Autodesk Fusion 360 part; units mm, degrees
(part 6 of 9)
  line L309 (-65.5897, 101.2894) -> (-69.9199, 98.7894)
  line L310 (-69.9199, 98.7894) -> (-74.25, 101.2894)
  line L311 (-74.25, 101.2894) -> (-74.25, 106.2894)
  line L312 (-48.8494, 97.4904) -> (-44.5192, 99.9904)
  line L313 (-44.5192, 99.9904) -> (-40.1891, 97.4904)
  line L314 (-40.1891, 97.4904) -> (-40.1891, 92.4904)
  line L315 (-40.1891, 92.4904) -> (-44.5192, 89.9904)
  line L316 (-44.5192, 89.9904) -> (-48.8494, 92.4904)
  line L317 (-48.8494, 92.4904) -> (-48.8494, 97.4904)
  line L318 (-23.4487, 88.6913) -> (-19.1186, 91.1913)
  line L319 (-19.1186, 91.1913) -> (-14.7885, 88.6913)
  line L320 (-14.7885, 88.6913) -> (-14.7885, 83.6913)
  line L321 (-14.7885, 83.6913) -> (-19.1186, 81.1913)
  line L322 (-19.1186, 81.1913) -> (-23.4487, 83.6913)
  line L323 (-23.4487, 83.6913) -> (-23.4487, 88.6913)
  line L324 (-64.0897, 88.6913) -> (-59.7596, 91.1913)
  line L325 (-59.7596, 91.1913) -> (-55.4295, 88.6913)
  line L326 (-55.4295, 88.6913) -> (-55.4295, 83.6913)
  line L327 (-55.4295, 83.6913) -> (-59.7596, 81.1913)
  line L328 (-59.7596, 81.1913) -> (-64.0897, 83.6913)
  line L329 (-64.0897, 83.6913) -> (-64.0897, 88.6913)
  line L330 (-38.6891, 79.8923) -> (-34.359, 82.3923)
  line L331 (-34.359, 82.3923) -> (-30.0289, 79.8923)
  line L332 (-30.0289, 79.8923) -> (-30.0289, 74.8923)
  line L333 (-30.0289, 74.8923) -> (-34.359, 72.3923)
  line L334 (-34.359, 72.3923) -> (-38.6891, 74.8923)
  line L335 (-38.6891, 74.8923) -> (-38.6891, 79.8923)
  line L336 (-79.3301, 79.8923) -> (-75, 82.3923)
  line L337 (-75, 82.3923) -> (-70.6699, 79.8923)
  line L338 (-70.6699, 79.8923) -> (-70.6699, 74.8923)
  line L339 (-70.6699, 74.8923) -> (-75, 72.3923)
  line L340 (-75, 72.3923) -> (-79.3301, 74.8923)
  line L341 (-79.3301, 74.8923) -> (-79.3301, 79.8923)
  line L342 (-53.9295, 71.0933) -> (-49.5994, 73.5933)
  line L343 (-49.5994, 73.5933) -> (-45.2692, 71.0933)
  line L344 (-45.2692, 71.0933) -> (-45.2692, 66.0933)
  line L345 (-45.2692, 66.0933) -> (-49.5994, 63.5933)
  line L346 (-49.5994, 63.5933) -> (-53.9295, 66.0933)
  line L347 (-53.9295, 66.0933) -> (-53.9295, 71.0933)
  line L348 (-28.5289, 62.2942) -> (-24.1987, 64.7942)
  line L349 (-24.1987, 64.7942) -> (-19.8686, 62.2942)
  line L350 (-19.8686, 62.2942) -> (-19.8686, 57.2942)
  line L351 (-19.8686, 57.2942) -> (-24.1987, 54.7942)
  line L352 (-24.1987, 54.7942) -> (-28.5289, 57.2942)
  line L353 (-28.5289, 57.2942) -> (-28.5289, 62.2942)
  line L354 (-69.1699, 62.2942) -> (-64.8397, 64.7942)
  line L355 (-64.8397, 64.7942) -> (-60.5096, 62.2942)
  line L356 (-60.5096, 62.2942) -> (-60.5096, 57.2942)
  line L357 (-60.5096, 57.2942) -> (-64.8397, 54.7942)
  line L358 (-64.8397, 54.7942) -> (-69.1699, 57.2942)
  line L359 (-69.1699, 57.2942) -> (-69.1699, 62.2942)
  line L360 (-43.7692, 53.4952) -> (-39.4391, 55.9952)
  line L361 (-39.4391, 55.9952) -> (-35.109, 53.4952)
  line L362 (-35.109, 53.4952) -> (-35.109, 48.4952)
  line L363 (-35.109, 48.4952) -> (-39.4391, 45.9952)
  line L364 (-39.4391, 45.9952) -> (-43.7692, 48.4952)
  line L365 (-43.7692, 48.4952) -> (-43.7692, 53.4952)
  line L366 (-18.3686, 44.6962) -> (-14.0385, 47.1962)
  line L367 (-14.0385, 47.1962) -> (-9.7083, 44.6962)
  line L368 (-9.7083, 44.6962) -> (-9.7083, 39.6962)
  line L369 (-9.7083, 39.6962) -> (-14.0385, 37.1962)
  line L370 (-14.0385, 37.1962) -> (-18.3686, 39.6962)
  line L371 (-18.3686, 39.6962) -> (-18.3686, 44.6962)
  line L372 (-59.0096, 44.6962) -> (-54.6795, 47.1962)
  line L373 (-54.6795, 47.1962) -> (-50.3494, 44.6962)
  line L374 (-50.3494, 44.6962) -> (-50.3494, 39.6962)
  line L375 (-50.3494, 39.6962) -> (-54.6795, 37.1962)
  line L376 (-54.6795, 37.1962) -> (-59.0096, 39.6962)
  line L377 (-59.0096, 39.6962) -> (-59.0096, 44.6962)
  line L378 (-33.609, 35.8971) -> (-29.2789, 38.3971)
  line L379 (-29.2789, 38.3971) -> (-24.9487, 35.8971)
  line L380 (-24.9487, 35.8971) -> (-24.9487, 30.8971)
  line L381 (-24.9487, 30.8971) -> (-29.2789, 28.3971)
  line L382 (-29.2789, 28.3971) -> (-33.609, 30.8971)
  line L383 (-33.609, 30.8971) -> (-33.609, 35.8971)
  line L384 (-74.25, 35.8971) -> (-69.9199, 38.3971)
  line L385 (-69.9199, 38.3971) -> (-65.5897, 35.8971)
  line L386 (-65.5897, 35.8971) -> (-65.5897, 30.8971)
  line L387 (-65.5897, 30.8971) -> (-69.9199, 28.3971)
  line L388 (-69.9199, 28.3971) -> (-74.25, 30.8971)
  line L389 (-74.25, 30.8971) -> (-74.25, 35.8971)
  line L390 (-48.8494, 27.0981) -> (-44.5192, 29.5981)
  line L391 (-44.5192, 29.5981) -> (-40.1891, 27.0981)
  line L392 (-40.1891, 27.0981) -> (-40.1891, 22.0981)
  line L393 (-40.1891, 22.0981) -> (-44.5192, 19.5981)
  line L394 (-44.5192, 19.5981) -> (-48.8494, 22.0981)
  line L395 (-48.8494, 22.0981) -> (-48.8494, 27.0981)
  line L396 (-23.4487, 18.299) -> (-19.1186, 20.799)
  line L397 (-19.1186, 20.799) -> (-14.7885, 18.299)
  line L398 (-14.7885, 18.299) -> (-14.7885, 13.299)
  line L399 (-14.7885, 13.299) -> (-19.1186, 10.799)
  line L400 (-19.1186, 10.799) -> (-23.4487, 13.299)
  line L401 (-23.4487, 13.299) -> (-23.4487, 18.299)
  line L402 (-64.0897, 18.299) -> (-59.7596, 20.799)
  line L403 (-59.7596, 20.799) -> (-55.4295, 18.299)
  line L404 (-55.4295, 18.299) -> (-55.4295, 13.299)
  line L405 (-55.4295, 13.299) -> (-59.7596, 10.799)
  line L406 (-59.7596, 10.799) -> (-64.0897, 13.299)
  line L407 (-64.0897, 13.299) -> (-64.0897, 18.299)
  line L408 (-53.9295, 18.299) -> (-49.5994, 20.799)
  line L409 (-49.5994, 20.799) -> (-45.2692, 18.299)
  line L410 (-45.2692, 18.299) -> (-45.2692, 13.299)
  line L411 (-45.2692, 13.299) -> (-49.5994, 10.799)
  line L412 (-49.5994, 10.799) -> (-53.9295, 13.299)
  line L413 (-53.9295, 13.299) -> (-53.9295, 18.299)
  line L414 (-79.3301, 27.0981) -> (-75, 29.5981)
  line L415 (-75, 29.5981) -> (-70.6699, 27.0981)
  line L416 (-70.6699, 27.0981) -> (-70.6699, 22.0981)
  line L417 (-70.6699, 22.0981) -> (-75, 19.5981)
  line L418 (-75, 19.5981) -> (-79.3301, 22.0981)
  line L419 (-79.3301, 22.0981) -> (-79.3301, 27.0981)
  line L420 (-38.6891, 27.0981) -> (-34.359, 29.5981)
  line L421 (-34.359, 29.5981) -> (-30.0289, 27.0981)
  line L422 (-30.0289, 27.0981) -> (-30.0289, 22.0981)
  line L423 (-30.0289, 22.0981) -> (-34.359, 19.5981)
  line L424 (-34.359, 19.5981) -> (-38.6891, 22.0981)
  line L425 (-38.6891, 22.0981) -> (-38.6891, 27.0981)
  line L426 (-64.0897, 35.8971) -> (-59.7596, 38.3971)
  line L427 (-59.7596, 38.3971) -> (-55.4295, 35.8971)
  line L428 (-55.4295, 35.8971) -> (-55.4295, 30.8971)
  line L429 (-55.4295, 30.8971) -> (-59.7596, 28.3971)
  line L430 (-59.7596, 28.3971) -> (-64.0897, 30.8971)
  line L431 (-64.0897, 30.8971) -> (-64.0897, 35.8971)
  line L432 (-23.4487, 35.8971) -> (-19.1186, 38.3971)
  line L433 (-19.1186, 38.3971) -> (-14.7885, 35.8971)
  line L434 (-14.7885, 35.8971) -> (-14.7885, 30.8971)
  line L435 (-14.7885, 30.8971) -> (-19.1186, 28.3971)
  line L436 (-19.1186, 28.3971) -> (-23.4487, 30.8971)
  line L437 (-23.4487, 30.8971) -> (-23.4487, 35.8971)
  line L438 (-48.8494, 44.6962) -> (-44.5192, 47.1962)
  line L439 (-44.5192, 47.1962) -> (-40.1891, 44.6962)
  line L440 (-40.1891, 44.6962) -> (-40.1891, 39.6962)
  line L441 (-40.1891, 39.6962) -> (-44.5192, 37.1962)
  line L442 (-44.5192, 37.1962) -> (-48.8494, 39.6962)
  line L443 (-48.8494, 39.6962) -> (-48.8494, 44.6962)
  line L444 (-74.25, 53.4952) -> (-69.9199, 55.9952)
  line L445 (-69.9199, 55.9952) -> (-65.5897, 53.4952)
  line L446 (-65.5897, 53.4952) -> (-65.5897, 48.4952)
  line L447 (-65.5897, 48.4952) -> (-69.9199, 45.9952)
  line L448 (-69.9199, 45.9952) -> (-74.25, 48.4952)
  line L449 (-74.25, 48.4952) -> (-74.25, 53.4952)
  line L450 (-33.609, 53.4952) -> (-29.2789, 55.9952)
  line L451 (-29.2789, 55.9952) -> (-24.9487, 53.4952)
  line L452 (-24.9487, 53.4952) -> (-24.9487, 48.4952)
  line L453 (-24.9487, 48.4952) -> (-29.2789, 45.9952)
  line L454 (-29.2789, 45.9952) -> (-33.609, 48.4952)
  line L455 (-33.609, 48.4952) -> (-33.609, 53.4952)
  line L456 (-59.0096, 62.2942) -> (-54.6795, 64.7942)
  line L457 (-54.6795, 64.7942) -> (-50.3494, 62.2942)
  line L458 (-50.3494, 62.2942) -> (-50.3494, 57.2942)
  line L459 (-50.3494, 57.2942) -> (-54.6795, 54.7942)
  line L460 (-54.6795, 54.7942) -> (-59.0096, 57.2942)
  line L461 (-59.0096, 57.2942) -> (-59.0096, 62.2942)
  line L462 (-18.3686, 62.2942) -> (-14.0385, 64.7942)
  line L463 (-14.0385, 64.7942) -> (-9.7083, 62.2942)
  line L464 (-9.7083, 62.2942) -> (-9.7083, 57.2942)
  line L465 (-9.7083, 57.2942) -> (-14.0385, 54.7942)
  line L466 (-14.0385, 54.7942) -> (-18.3686, 57.2942)
  line L467 (-18.3686, 57.2942) -> (-18.3686, 62.2942)
  line L468 (-43.7692, 71.0933) -> (-39.4391, 73.5933)
  line L469 (-39.4391, 73.5933) -> (-35.109, 71.0933)
  line L470 (-35.109, 71.0933) -> (-35.109, 66.0933)
  line L471 (-35.109, 66.0933) -> (-39.4391, 63.5933)
  line L472 (-39.4391, 63.5933) -> (-43.7692, 66.0933)
  line L473 (-43.7692, 66.0933) -> (-43.7692, 71.0933)
  line L474 (-69.1699, 79.8923) -> (-64.8397, 82.3923)
  line L475 (-64.8397, 82.3923) -> (-60.5096, 79.8923)
  line L476 (-60.5096, 79.8923) -> (-60.5096, 74.8923)
  line L477 (-60.5096, 74.8923) -> (-64.8397, 72.3923)
  line L478 (-64.8397, 72.3923) -> (-69.1699, 74.8923)
  line L479 (-69.1699, 74.8923) -> (-69.1699, 79.8923)
  line L480 (-28.5289, 79.8923) -> (-24.1987, 82.3923)
  line L481 (-24.1987, 82.3923) -> (-19.8686, 79.8923)
  line L482 (-19.8686, 79.8923) -> (-19.8686, 74.8923)
  line L483 (-19.8686, 74.8923) -> (-24.1987, 72.3923)
  line L484 (-24.1987, 72.3923) -> (-28.5289, 74.8923)
  line L485 (-28.5289, 74.8923) -> (-28.5289, 79.8923)
  line L486 (-53.9295, 88.6913) -> (-49.5994, 91.1913)
  line L487 (-49.5994, 91.1913) -> (-45.2692, 88.6913)
  line L488 (-45.2692, 88.6913) -> (-45.2692, 83.6913)
  line L489 (-45.2692, 83.6913) -> (-49.5994, 81.1913)
  line L490 (-49.5994, 81.1913) -> (-53.9295, 83.6913)
  line L491 (-53.9295, 83.6913) -> (-53.9295, 88.6913)
  line L492 (-79.3301, 97.4904) -> (-75, 99.9904)
  line L493 (-75, 99.9904) -> (-70.6699, 97.4904)
  line L494 (-70.6699, 97.4904) -> (-70.6699, 92.4904)
  line L495 (-70.6699, 92.4904) -> (-75, 89.9904)
  line L496 (-75, 89.9904) -> (-79.3301, 92.4904)
  line L497 (-79.3301, 92.4904) -> (-79.3301, 97.4904)
  line L498 (-38.6891, 97.4904) -> (-34.359, 99.9904)
  line L499 (-34.359, 99.9904) -> (-30.0289, 97.4904)
  line L500 (-30.0289, 97.4904) -> (-30.0289, 92.4904)
  line L501 (-30.0289, 92.4904) -> (-34.359, 89.9904)
  line L502 (-34.359, 89.9904) -> (-38.6891, 92.4904)
  line L503 (-38.6891, 92.4904) -> (-38.6891, 97.4904)
  line L504 (-64.0897, 106.2894) -> (-59.7596, 108.7894)
  line L505 (-59.7596, 108.7894) -> (-55.4295, 106.2894)
  line L506 (-55.4295, 106.2894) -> (-55.4295, 101.2894)
  line L507 (-55.4295, 101.2894) -> (-59.7596, 98.7894)
  line L508 (-59.7596, 98.7894) -> (-64.0897, 101.2894)
  line L509 (-64.0897, 101.2894) -> (-64.0897, 106.2894)
  line L510 (-23.4487, 106.2894) -> (-19.1186, 108.7894)
  line L511 (-19.1186, 108.7894) -> (-14.7885, 106.2894)
  line L512 (-14.7885, 106.2894) -> (-14.7885, 101.2894)
  line L513 (-14.7885, 101.2894) -> (-19.1186, 98.7894)
  line L514 (-19.1186, 98.7894) -> (-23.4487, 101.2894)
  line L515 (-23.4487, 101.2894) -> (-23.4487, 106.2894)
  line L516 (-48.8494, 115.0885) -> (-44.5192, 117.5885)
  line L517 (-44.5192, 117.5885) -> (-40.1891, 115.0885)
  line L518 (-40.1891, 115.0885) -> (-40.1891, 110.0885)
  line L519 (-40.1891, 110.0885) -> (-44.5192, 107.5885)
  line L520 (-44.5192, 107.5885) -> (-48.8494, 110.0885)
  line L521 (-48.8494, 110.0885) -> (-48.8494, 115.0885)
  line L522 (-74.25, 123.8875) -> (-69.9199, 126.3875)
  line L523 (-69.9199, 126.3875) -> (-65.5897, 123.8875)
  line L524 (-65.5897, 123.8875) -> (-65.5897, 118.8875)
  line L525 (-65.5897, 118.8875) -> (-69.9199, 116.3875)
  line L526 (-69.9199, 116.3875) -> (-74.25, 118.8875)
  line L527 (-74.25, 118.8875) -> (-74.25, 123.8875)
  line L528 (-33.609, 123.8875) -> (-29.2789, 126.3875)
  line L529 (-29.2789, 126.3875) -> (-24.9487, 123.8875)
  line L530 (-24.9487, 123.8875) -> (-24.9487, 118.8875)
  line L531 (-24.9487, 118.8875) -> (-29.2789, 116.3875)
  line L532 (-29.2789, 116.3875) -> (-33.609, 118.8875)
  line L533 (-33.609, 118.8875) -> (-33.609, 123.8875)
  line L534 (-59.0096, 132.6865) -> (-54.6795, 135.1865)
  line L535 (-54.6795, 135.1865) -> (-50.3494, 132.6865)
  line L536 (-50.3494, 132.6865) -> (-50.3494, 127.6865)
  line L537 (-50.3494, 127.6865) -> (-54.6795, 125.1865)
  line L538 (-54.6795, 125.1865) -> (-59.0096, 127.6865)
  line L539 (-59.0096, 127.6865) -> (-59.0096, 132.6865)
  line L540 (-18.3686, 132.6865) -> (-14.0385, 135.1865)
  line L541 (-14.0385, 135.1865) -> (-9.7083, 132.6865)
  line L542 (-9.7083, 132.6865) -> (-9.7083, 127.6865)
  line L543 (-9.7083, 127.6865) -> (-14.0385, 125.1865)
  line L544 (-14.0385, 125.1865) -> (-18.3686, 127.6865)
  line L545 (-18.3686, 127.6865) -> (-18.3686, 132.6865)
  line L546 (-82, 0) -> (-7, 0)
  line L547 (-7, 0) -> (-7, 140)
  line L548 (-7, 140) -> (-82, 140)
  line L549 (-82, 140) -> (-82, 0)
  line L550 (-69.9199, 20.799) -> (-74.25, 18.299)
  line L551 (-74.25, 18.299) -> (-74.25, 13.299)
  line L552 (-74.25, 13.299) -> (-69.9199, 10.799)
  line L553 (-69.9199, 10.799) -> (-65.5897, 13.299)
  line L554 (-65.5897, 13.299) -> (-65.5897, 18.299)
  line L555 (-65.5897, 18.299) -> (-69.9199, 20.799)
  line L556 (-59.7596, 20.799) -> (-64.0897, 18.299)
  line L557 (-64.0897, 18.299) -> (-64.0897, 13.299)
  line L558 (-64.0897, 13.299) -> (-59.7596, 10.799)
  line L559 (-59.7596, 10.799) -> (-55.4295, 13.299)
  line L560 (-55.4295, 13.299) -> (-55.4295, 18.299)
  line L561 (-55.4295, 18.299) -> (-59.7596, 20.799)
  line L562 (-49.5994, 20.799) -> (-53.9295, 18.299)
  line L563 (-53.9295, 18.299) -> (-53.9295, 13.299)
  line L564 (-53.9295, 13.299) -> (-49.5994, 10.799)
  line L565 (-49.5994, 10.799) -> (-45.2692, 13.299)
  line L566 (-45.2692, 13.299) -> (-45.2692, 18.299)
  line L567 (-45.2692, 18.299) -> (-49.5994, 20.799)
  line L568 (-39.4391, 20.799) -> (-43.7692, 18.299)
  line L569 (-43.7692, 18.299) -> (-43.7692, 13.299)
  line L570 (-43.7692, 13.299) -> (-39.4391, 10.799)
  line L571 (-39.4391, 10.799) -> (-35.109, 13.299)
  line L572 (-35.109, 13.299) -> (-35.109, 18.299)
  line L573 (-35.109, 18.299) -> (-39.4391, 20.799)
  line L574 (-29.2789, 20.799) -> (-33.609, 18.299)
  line L575 (-33.609, 18.299) -> (-33.609, 13.299)
  line L576 (-33.609, 13.299) -> (-29.2789, 10.799)
  line L577 (-29.2789, 10.799) -> (-24.9487, 13.299)
  line L578 (-24.9487, 13.299) -> (-24.9487, 18.299)
  line L579 (-24.9487, 18.299) -> (-29.2789, 20.799)
  line L580 (-19.1186, 20.799) -> (-23.4487, 18.299)
  line L581 (-23.4487, 18.299) -> (-23.4487, 13.299)
  line L582 (-23.4487, 13.299) -> (-19.1186, 10.799)
  line L583 (-19.1186, 10.799) -> (-14.7885, 13.299)
  line L584 (-14.7885, 13.299) -> (-14.7885, 18.299)
  line L585 (-14.7885, 18.299) -> (-19.1186, 20.799)
  line L586 (-75, 29.5981) -> (-79.3301, 27.0981)
  line L587 (-79.3301, 27.0981) -> (-79.3301, 22.0981)
  line L588 (-79.3301, 22.0981) -> (-75, 19.5981)
  line L589 (-75, 19.5981) -> (-70.6699, 22.0981)
  line L590 (-70.6699, 22.0981) -> (-70.6699, 27.0981)
  line L591 (-70.6699, 27.0981) -> (-75, 29.5981)
  line L592 (-64.8397, 29.5981) -> (-69.1699, 27.0981)
  line L593 (-69.1699, 27.0981) -> (-69.1699, 22.0981)
  line L594 (-69.1699, 22.0981) -> (-64.8397, 19.5981)
  line L595 (-64.8397, 19.5981) -> (-60.5096, 22.0981)
  line L596 (-60.5096, 22.0981) -> (-60.5096, 27.0981)
  line L597 (-60.5096, 27.0981) -> (-64.8397, 29.5981)
  line L598 (-54.6795, 29.5981) -> (-59.0096, 27.0981)
  line L599 (-59.0096, 27.0981) -> (-59.0096, 22.0981)
  line L600 (-59.0096, 22.0981) -> (-54.6795, 19.5981)
  line L601 (-54.6795, 19.5981) -> (-50.3494, 22.0981)
  line L602 (-50.3494, 22.0981) -> (-50.3494, 27.0981)
  line L603 (-50.3494, 27.0981) -> (-54.6795, 29.5981)
  line L604 (-44.5192, 29.5981) -> (-48.8494, 27.0981)
  line L605 (-48.8494, 27.0981) -> (-48.8494, 22.0981)
  line L606 (-48.8494, 22.0981) -> (-44.5192, 19.5981)
  line L607 (-44.5192, 19.5981) -> (-40.1891, 22.0981)
  line L608 (-40.1891, 22.0981) -> (-40.1891, 27.0981)
  line L609 (-40.1891, 27.0981) -> (-44.5192, 29.5981)
  line L610 (-34.359, 29.5981) -> (-38.6891, 27.0981)
  line L611 (-38.6891, 27.0981) -> (-38.6891, 22.0981)
  line L612 (-38.6891, 22.0981) -> (-34.359, 19.5981)
  line L613 (-34.359, 19.5981) -> (-30.0289, 22.0981)
  line L614 (-30.0289, 22.0981) -> (-30.0289, 27.0981)
  line L615 (-30.0289, 27.0981) -> (-34.359, 29.5981)
  line L616 (-24.1987, 29.5981) -> (-28.5289, 27.0981)
  line L617 (-28.5289, 27.0981) -> (-28.5289, 22.0981)
  line L618 (-28.5289, 22.0981) -> (-24.1987, 19.5981)
  line L619 (-24.1987, 19.5981) -> (-19.8686, 22.0981)
  line L620 (-19.8686, 22.0981) -> (-19.8686, 27.0981)
  line L621 (-19.8686, 27.0981) -> (-24.1987, 29.5981)
  line L622 (-14.0385, 29.5981) -> (-18.3686, 27.0981)
  line L623 (-18.3686, 27.0981) -> (-18.3686, 22.0981)
  line L624 (-18.3686, 22.0981) -> (-14.0385, 19.5981)
  line L625 (-14.0385, 19.5981) -> (-9.7083, 22.0981)
  line L626 (-9.7083, 22.0981) -> (-9.7083, 27.0981)
  line L627 (-9.7083, 27.0981) -> (-14.0385, 29.5981)
  line L628 (-69.9199, 38.3971) -> (-74.25, 35.8971)
  line L629 (-74.25, 35.8971) -> (-74.25, 30.8971)
  line L630 (-74.25, 30.8971) -> (-69.9199, 28.3971)
  line L631 (-69.9199, 28.3971) -> (-65.5897, 30.8971)
  line L632 (-65.5897, 30.8971) -> (-65.5897, 35.8971)
  line L633 (-65.5897, 35.8971) -> (-69.9199, 38.3971)
  line L634 (-59.7596, 38.3971) -> (-64.0897, 35.8971)
  line L635 (-64.0897, 35.8971) -> (-64.0897, 30.8971)
  line L636 (-64.0897, 30.8971) -> (-59.7596, 28.3971)
  line L637 (-59.7596, 28.3971) -> (-55.4295, 30.8971)
  line L638 (-55.4295, 30.8971) -> (-55.4295, 35.8971)
  line L639 (-55.4295, 35.8971) -> (-59.7596, 38.3971)
  line L640 (-49.5994, 38.3971) -> (-53.9295, 35.8971)
  line L641 (-53.9295, 35.8971) -> (-53.9295, 30.8971)
  line L642 (-53.9295, 30.8971) -> (-49.5994, 28.3971)
  line L643 (-49.5994, 28.3971) -> (-45.2692, 30.8971)
  line L644 (-45.2692, 30.8971) -> (-45.2692, 35.8971)
  line L645 (-45.2692, 35.8971) -> (-49.5994, 38.3971)
  line L646 (-39.4391, 38.3971) -> (-43.7692, 35.8971)
  line L647 (-43.7692, 35.8971) -> (-43.7692, 30.8971)
  line L648 (-43.7692, 30.8971) -> (-39.4391, 28.3971)
  line L649 (-39.4391, 28.3971) -> (-35.109, 30.8971)
  line L650 (-35.109, 30.8971) -> (-35.109, 35.8971)
  line L651 (-35.109, 35.8971) -> (-39.4391, 38.3971)
  line L652 (-29.2789, 38.3971) -> (-33.609, 35.8971)
  line L653 (-33.609, 35.8971) -> (-33.609, 30.8971)
  line L654 (-33.609, 30.8971) -> (-29.2789, 28.3971)
  line L655 (-29.2789, 28.3971) -> (-24.9487, 30.8971)
  line L656 (-24.9487, 30.8971) -> (-24.9487, 35.8971)
  line L657 (-24.9487, 35.8971) -> (-29.2789, 38.3971)
  line L658 (-19.1186, 38.3971) -> (-23.4487, 35.8971)
  line L659 (-23.4487, 35.8971) -> (-23.4487, 30.8971)
  line L660 (-23.4487, 30.8971) -> (-19.1186, 28.3971)
  line L661 (-19.1186, 28.3971) -> (-14.7885, 30.8971)
  line L662 (-14.7885, 30.8971) -> (-14.7885, 35.8971)
  line L663 (-14.7885, 35.8971) -> (-19.1186, 38.3971)
  line L664 (-75, 47.1962) -> (-79.3301, 44.6962)
  line L665 (-79.3301, 44.6962) -> (-79.3301, 39.6962)
  line L666 (-79.3301, 39.6962) -> (-75, 37.1962)
  line L667 (-75, 37.1962) -> (-70.6699, 39.6962)
  line L668 (-70.6699, 39.6962) -> (-70.6699, 44.6962)
  line L669 (-70.6699, 44.6962) -> (-75, 47.1962)
  line L670 (-64.8397, 47.1962) -> (-69.1699, 44.6962)
  line L671 (-69.1699, 44.6962) -> (-69.1699, 39.6962)
  line L672 (-69.1699, 39.6962) -> (-64.8397, 37.1962)
  line L673 (-64.8397, 37.1962) -> (-60.5096, 39.6962)
  line L674 (-60.5096, 39.6962) -> (-60.5096, 44.6962)
  line L675 (-60.5096, 44.6962) -> (-64.8397, 47.1962)
  line L676 (-54.6795, 47.1962) -> (-59.0096, 44.6962)
  line L677 (-59.0096, 44.6962) -> (-59.0096, 39.6962)
  line L678 (-59.0096, 39.6962) -> (-54.6795, 37.1962)
  line L679 (-54.6795, 37.1962) -> (-50.3494, 39.6962)
  line L680 (-50.3494, 39.6962) -> (-50.3494, 44.6962)
  line L681 (-50.3494, 44.6962) -> (-54.6795, 47.1962)
  line L682 (-44.5192, 47.1962) -> (-48.8494, 44.6962)
  line L683 (-48.8494, 44.6962) -> (-48.8494, 39.6962)
  line L684 (-48.8494, 39.6962) -> (-44.5192, 37.1962)
  line L685 (-44.5192, 37.1962) -> (-40.1891, 39.6962)
  line L686 (-40.1891, 39.6962) -> (-40.1891, 44.6962)
  line L687 (-40.1891, 44.6962) -> (-44.5192, 47.1962)
  line L688 (-34.359, 47.1962) -> (-38.6891, 44.6962)
  line L689 (-38.6891, 44.6962) -> (-38.6891, 39.6962)
  line L690 (-38.6891, 39.6962) -> (-34.359, 37.1962)
  line L691 (-34.359, 37.1962) -> (-30.0289, 39.6962)
  line L692 (-30.0289, 39.6962) -> (-30.0289, 44.6962)
  line L693 (-30.0289, 44.6962) -> (-34.359, 47.1962)
  line L694 (-24.1987, 47.1962) -> (-28.5289, 44.6962)
  line L695 (-28.5289, 44.6962) -> (-28.5289, 39.6962)
  line L696 (-28.5289, 39.6962) -> (-24.1987, 37.1962)
  line L697 (-24.1987, 37.1962) -> (-19.8686, 39.6962)
  line L698 (-19.8686, 39.6962) -> (-19.8686, 44.6962)
  line L699 (-19.8686, 44.6962) -> (-24.1987, 47.1962)
  line L700 (-14.0385, 47.1962) -> (-18.3686, 44.6962)
  line L701 (-18.3686, 44.6962) -> (-18.3686, 39.6962)
  line L702 (-18.3686, 39.6962) -> (-14.0385, 37.1962)
  line L703 (-14.0385, 37.1962) -> (-9.7083, 39.6962)
  line L704 (-9.7083, 39.6962) -> (-9.7083, 44.6962)
  line L705 (-9.7083, 44.6962) -> (-14.0385, 47.1962)
  line L706 (-69.9199, 55.9952) -> (-74.25, 53.4952)
  line L707 (-74.25, 53.4952) -> (-74.25, 48.4952)
  line L708 (-74.25, 48.4952) -> (-69.9199, 45.9952)
  line L709 (-69.9199, 45.9952) -> (-65.5897, 48.4952)
  line L710 (-65.5897, 48.4952) -> (-65.5897, 53.4952)
  line L711 (-65.5897, 53.4952) -> (-69.9199, 55.9952)
  line L712 (-59.7596, 55.9952) -> (-64.0897, 53.4952)
  line L713 (-64.0897, 53.4952) -> (-64.0897, 48.4952)
  line L714 (-64.0897, 48.4952) -> (-59.7596, 45.9952)
  line L715 (-59.7596, 45.9952) -> (-55.4295, 48.4952)
  line L716 (-55.4295, 48.4952) -> (-55.4295, 53.4952)
  line L717 (-55.4295, 53.4952) -> (-59.7596, 55.9952)
  line L718 (-49.5994, 55.9952) -> (-53.9295, 53.4952)
  line L719 (-53.9295, 53.4952) -> (-53.9295, 48.4952)
  line L720 (-53.9295, 48.4952) -> (-49.5994, 45.9952)
  line L721 (-49.5994, 45.9952) -> (-45.2692, 48.4952)
  line L722 (-45.2692, 48.4952) -> (-45.2692, 53.4952)
  line L723 (-45.2692, 53.4952) -> (-49.5994, 55.9952)
  line L724 (-39.4391, 55.9952) -> (-43.7692, 53.4952)
  line L725 (-43.7692, 53.4952) -> (-43.7692, 48.4952)
  line L726 (-43.7692, 48.4952) -> (-39.4391, 45.9952)
  line L727 (-39.4391, 45.9952) -> (-35.109, 48.4952)
  line L728 (-35.109, 48.4952) -> (-35.109, 53.4952)
  line L729 (-35.109, 53.4952) -> (-39.4391, 55.9952)
  line L730 (-29.2789, 55.9952) -> (-33.609, 53.4952)
  line L731 (-33.609, 53.4952) -> (-33.609, 48.4952)
  line L732 (-33.609, 48.4952) -> (-29.2789, 45.9952)
  line L733 (-29.2789, 45.9952) -> (-24.9487, 48.4952)
  line L734 (-24.9487, 48.4952) -> (-24.9487, 53.4952)
  line L735 (-24.9487, 53.4952) -> (-29.2789, 55.9952)
  line L736 (-19.1186, 55.9952) -> (-23.4487, 53.4952)
  line L737 (-23.4487, 53.4952) -> (-23.4487, 48.4952)
  line L738 (-23.4487, 48.4952) -> (-19.1186, 45.9952)
  line L739 (-19.1186, 45.9952) -> (-14.7885, 48.4952)
  line L740 (-14.7885, 48.4952) -> (-14.7885, 53.4952)
  line L741 (-14.7885, 53.4952) -> (-19.1186, 55.9952)
  line L742 (-75, 64.7942) -> (-79.3301, 62.2942)
  line L743 (-79.3301, 62.2942) -> (-79.3301, 57.2942)
  line L744 (-79.3301, 57.2942) -> (-75, 54.7942)
  line L745 (-75, 54.7942) -> (-70.6699, 57.2942)
  line L746 (-70.6699, 57.2942) -> (-70.6699, 62.2942)
  line L747 (-70.6699, 62.2942) -> (-75, 64.7942)
  line L748 (-64.8397, 64.7942) -> (-69.1699, 62.2942)
  line L749 (-69.1699, 62.2942) -> (-69.1699, 57.2942)
  line L750 (-69.1699, 57.2942) -> (-64.8397, 54.7942)
  line L751 (-64.8397, 54.7942) -> (-60.5096, 57.2942)
  line L752 (-60.5096, 57.2942) -> (-60.5096, 62.2942)
  line L753 (-60.5096, 62.2942) -> (-64.8397, 64.7942)
  line L754 (-54.6795, 64.7942) -> (-59.0096, 62.2942)
  line L755 (-59.0096, 62.2942) -> (-59.0096, 57.2942)
  line L756 (-59.0096, 57.2942) -> (-54.6795, 54.7942)
  line L757 (-54.6795, 54.7942) -> (-50.3494, 57.2942)
  line L758 (-50.3494, 57.2942) -> (-50.3494, 62.2942)
  line L759 (-50.3494, 62.2942) -> (-54.6795, 64.7942)
  line L760 (-44.5192, 64.7942) -> (-48.8494, 62.2942)
  line L761 (-48.8494, 62.2942) -> (-48.8494, 57.2942)
  line L762 (-48.8494, 57.2942) -> (-44.5192, 54.7942)
  line L763 (-44.5192, 54.7942) -> (-40.1891, 57.2942)
  line L764 (-40.1891, 57.2942) -> (-40.1891, 62.2942)
  line L765 (-40.1891, 62.2942) -> (-44.5192, 64.7942)
  line L766 (-34.359, 64.7942) -> (-38.6891, 62.2942)
  line L767 (-38.6891, 62.2942) -> (-38.6891, 57.2942)
  line L768 (-38.6891, 57.2942) -> (-34.359, 54.7942)
  line L769 (-34.359, 54.7942) -> (-30.0289, 57.2942)
  line L770 (-30.0289, 57.2942) -> (-30.0289, 62.2942)
  line L771 (-30.0289, 62.2942) -> (-34.359, 64.7942)
  line L772 (-24.1987, 64.7942) -> (-28.5289, 62.2942)
  line L773 (-28.5289, 62.2942) -> (-28.5289, 57.2942)
  line L774 (-28.5289, 57.2942) -> (-24.1987, 54.7942)
  line L775 (-24.1987, 54.7942) -> (-19.8686, 57.2942)
  line L776 (-19.8686, 57.2942) -> (-19.8686, 62.2942)
  line L777 (-19.8686, 62.2942) -> (-24.1987, 64.7942)
  line L778 (-14.0385, 64.7942) -> (-18.3686, 62.2942)
  line L779 (-18.3686, 62.2942) -> (-18.3686, 57.2942)
  line L780 (-18.3686, 57.2942) -> (-14.0385, 54.7942)
  line L781 (-14.0385, 54.7942) -> (-9.7083, 57.2942)
  line L782 (-9.7083, 57.2942) -> (-9.7083, 62.2942)
  line L783 (-9.7083, 62.2942) -> (-14.0385, 64.7942)
  line L784 (-69.9199, 73.5933) -> (-74.25, 71.0933)
  line L785 (-74.25, 71.0933) -> (-74.25, 66.0933)
  line L786 (-74.25, 66.0933) -> (-69.9199, 63.5933)
  line L787 (-69.9199, 63.5933) -> (-65.5897, 66.0933)
  line L788 (-65.5897, 66.0933) -> (-65.5897, 71.0933)
  line L789 (-65.5897, 71.0933) -> (-69.9199, 73.5933)
  line L790 (-59.7596, 73.5933) -> (-64.0897, 71.0933)
  line L791 (-64.0897, 71.0933) -> (-64.0897, 66.0933)
  line L792 (-64.0897, 66.0933) -> (-59.7596, 63.5933)
  line L793 (-59.7596, 63.5933) -> (-55.4295, 66.0933)
  line L794 (-55.4295, 66.0933) -> (-55.4295, 71.0933)
  line L795 (-55.4295, 71.0933) -> (-59.7596, 73.5933)
  line L796 (-49.5994, 73.5933) -> (-53.9295, 71.0933)
  line L797 (-53.9295, 71.0933) -> (-53.9295, 66.0933)
  line L798 (-53.9295, 66.0933) -> (-49.5994, 63.5933)
  line L799 (-49.5994, 63.5933) -> (-45.2692, 66.0933)
  line L800 (-45.2692, 66.0933) -> (-45.2692, 71.0933)
  line L801 (-45.2692, 71.0933) -> (-49.5994, 73.5933)
  line L802 (-39.4391, 73.5933) -> (-43.7692, 71.0933)
  line L803 (-43.7692, 71.0933) -> (-43.7692, 66.0933)
  line L804 (-43.7692, 66.0933) -> (-39.4391, 63.5933)
  line L805 (-39.4391, 63.5933) -> (-35.109, 66.0933)
  line L806 (-35.109, 66.0933) -> (-35.109, 71.0933)
  line L807 (-35.109, 71.0933) -> (-39.4391, 73.5933)
  line L808 (-29.2789, 73.5933) -> (-33.609, 71.0933)
  line L809 (-33.609, 71.0933) -> (-33.609, 66.0933)
  line L810 (-33.609, 66.0933) -> (-29.2789, 63.5933)
  line L811 (-29.2789, 63.5933) -> (-24.9487, 66.0933)
  line L812 (-24.9487, 66.0933) -> (-24.9487, 71.0933)
  line L813 (-24.9487, 71.0933) -> (-29.2789, 73.5933)
  line L814 (-19.1186, 73.5933) -> (-23.4487, 71.0933)
  line L815 (-23.4487, 71.0933) -> (-23.4487, 66.0933)
  line L816 (-23.4487, 66.0933) -> (-19.1186, 63.5933)
  line L817 (-19.1186, 63.5933) -> (-14.7885, 66.0933)
  line L818 (-14.7885, 66.0933) -> (-14.7885, 71.0933)
  line L819 (-14.7885, 71.0933) -> (-19.1186, 73.5933)
  line L820 (-75, 82.3923) -> (-79.3301, 79.8923)
  line L821 (-79.3301, 79.8923) -> (-79.3301, 74.8923)
  line L822 (-79.3301, 74.8923) -> (-75, 72.3923)
  line L823 (-75, 72.3923) -> (-70.6699, 74.8923)
  line L824 (-70.6699, 74.8923) -> (-70.6699, 79.8923)
  line L825 (-70.6699, 79.8923) -> (-75, 82.3923)
  line L826 (-64.8397, 82.3923) -> (-69.1699, 79.8923)
  line L827 (-69.1699, 79.8923) -> (-69.1699, 74.8923)
  line L828 (-69.1699, 74.8923) -> (-64.8397, 72.3923)
  line L829 (-64.8397, 72.3923) -> (-60.5096, 74.8923)
  line L830 (-60.5096, 74.8923) -> (-60.5096, 79.8923)
  line L831 (-60.5096, 79.8923) -> (-64.8397, 82.3923)
  line L832 (-54.6795, 82.3923) -> (-59.0096, 79.8923)
  line L833 (-59.0096, 79.8923) -> (-59.0096, 74.8923)
  line L834 (-59.0096, 74.8923) -> (-54.6795, 72.3923)
  line L835 (-54.6795, 72.3923) -> (-50.3494, 74.8923)
  line L836 (-50.3494, 74.8923) -> (-50.3494, 79.8923)
  line L837 (-50.3494, 79.8923) -> (-54.6795, 82.3923)
  line L838 (-44.5192, 82.3923) -> (-48.8494, 79.8923)
  line L839 (-48.8494, 79.8923) -> (-48.8494, 74.8923)
  line L840 (-48.8494, 74.8923) -> (-44.5192, 72.3923)
  line L841 (-44.5192, 72.3923) -> (-40.1891, 74.8923)
  line L842 (-40.1891, 74.8923) -> (-40.1891, 79.8923)
  line L843 (-40.1891, 79.8923) -> (-44.5192, 82.3923)
  line L844 (-34.359, 82.3923) -> (-38.6891, 79.8923)
  line L845 (-38.6891, 79.8923) -> (-38.6891, 74.8923)
  line L846 (-38.6891, 74.8923) -> (-34.359, 72.3923)
  line L847 (-34.359, 72.3923) -> (-30.0289, 74.8923)
  line L848 (-30.0289, 74.8923) -> (-30.0289, 79.8923)
  line L849 (-30.0289, 79.8923) -> (-34.359, 82.3923)
  line L850 (-24.1987, 82.3923) -> (-28.5289, 79.8923)
  line L851 (-28.5289, 79.8923) -> (-28.5289, 74.8923)
  line L852 (-28.5289, 74.8923) -> (-24.1987, 72.3923)
  line L853 (-24.1987, 72.3923) -> (-19.8686, 74.8923)
  line L854 (-19.8686, 74.8923) -> (-19.8686, 79.8923)
  line L855 (-19.8686, 79.8923) -> (-24.1987, 82.3923)
  line L856 (-14.0385, 82.3923) -> (-18.3686, 79.8923)
  line L857 (-18.3686, 79.8923) -> (-18.3686, 74.8923)
  line L858 (-18.3686, 74.8923) -> (-14.0385, 72.3923)
  line L859 (-14.0385, 72.3923) -> (-9.7083, 74.8923)
  line L860 (-9.7083, 74.8923) -> (-9.7083, 79.8923)
  line L861 (-9.7083, 79.8923) -> (-14.0385, 82.3923)
  line L862 (-69.9199, 91.1913) -> (-74.25, 88.6913)
  line L863 (-74.25, 88.6913) -> (-74.25, 83.6913)
  line L864 (-74.25, 83.6913) -> (-69.9199, 81.1913)
  line L865 (-69.9199, 81.1913) -> (-65.5897, 83.6913)
  line L866 (-65.5897, 83.6913) -> (-65.5897, 88.6913)
  line L867 (-65.5897, 88.6913) -> (-69.9199, 91.1913)
  line L868 (-59.7596, 91.1913) -> (-64.0897, 88.6913)
  line L869 (-64.0897, 88.6913) -> (-64.0897, 83.6913)
  line L870 (-64.0897, 83.6913) -> (-59.7596, 81.1913)
  line L871 (-59.7596, 81.1913) -> (-55.4295, 83.6913)
  line L872 (-55.4295, 83.6913) -> (-55.4295, 88.6913)
  line L873 (-55.4295, 88.6913) -> (-59.7596, 91.1913)
  line L874 (-49.5994, 91.1913) -> (-53.9295, 88.6913)
  line L875 (-53.9295, 88.6913) -> (-53.9295, 83.6913)
  line L876 (-53.9295, 83.6913) -> (-49.5994, 81.1913)
  line L877 (-49.5994, 81.1913) -> (-45.2692, 83.6913)
  line L878 (-45.2692, 83.6913) -> (-45.2692, 88.6913)
  line L879 (-45.2692, 88.6913) -> (-49.5994, 91.1913)
  line L880 (-39.4391, 91.1913) -> (-43.7692, 88.6913)
  line L881 (-43.7692, 88.6913) -> (-43.7692, 83.6913)
  line L882 (-43.7692, 83.6913) -> (-39.4391, 81.1913)
  line L883 (-39.4391, 81.1913) -> (-35.109, 83.6913)
  line L884 (-35.109, 83.6913) -> (-35.109, 88.6913)
  line L885 (-35.109, 88.6913) -> (-39.4391, 91.1913)
  line L886 (-29.2789, 91.1913) -> (-33.609, 88.6913)
  line L887 (-33.609, 88.6913) -> (-33.609, 83.6913)
  line L888 (-33.609, 83.6913) -> (-29.2789, 81.1913)
  line L889 (-29.2789, 81.1913) -> (-24.9487, 83.6913)
  line L890 (-24.9487, 83.6913) -> (-24.9487, 88.6913)
  line L891 (-24.9487, 88.6913) -> (-29.2789, 91.1913)
  line L892 (-19.1186, 91.1913) -> (-23.4487, 88.6913)
  line L893 (-23.4487, 88.6913) -> (-23.4487, 83.6913)
  line L894 (-23.4487, 83.6913) -> (-19.1186, 81.1913)
  line L895 (-19.1186, 81.1913) -> (-14.7885, 83.6913)
  line L896 (-14.7885, 83.6913) -> (-14.7885, 88.6913)
  line L897 (-14.7885, 88.6913) -> (-19.1186, 91.1913)
  line L898 (-75, 99.9904) -> (-79.3301, 97.4904)
  line L899 (-79.3301, 97.4904) -> (-79.3301, 92.4904)
  line L900 (-79.3301, 92.4904) -> (-75, 89.9904)
  line L901 (-75, 89.9904) -> (-70.6699, 92.4904)
  line L902 (-70.6699, 92.4904) -> (-70.6699, 97.4904)
  line L903 (-70.6699, 97.4904) -> (-75, 99.9904)
  line L904 (-64.8397, 99.9904) -> (-69.1699, 97.4904)
  line L905 (-69.1699, 97.4904) -> (-69.1699, 92.4904)
  line L906 (-69.1699, 92.4904) -> (-64.8397, 89.9904)
  line L907 (-64.8397, 89.9904) -> (-60.5096, 92.4904)
  line L908 (-60.5096, 92.4904) -> (-60.5096, 97.4904)
  line L909 (-60.5096, 97.4904) -> (-64.8397, 99.9904)
  line L910 (-54.6795, 99.9904) -> (-59.0096, 97.4904)
  line L911 (-59.0096, 97.4904) -> (-59.0096, 92.4904)
  line L912 (-59.0096, 92.4904) -> (-54.6795, 89.9904)
  line L913 (-54.6795, 89.9904) -> (-50.3494, 92.4904)
  line L914 (-50.3494, 92.4904) -> (-50.3494, 97.4904)
  line L915 (-50.3494, 97.4904) -> (-54.6795, 99.9904)
  line L916 (-44.5192, 99.9904) -> (-48.8494, 97.4904)
  line L917 (-48.8494, 97.4904) -> (-48.8494, 92.4904)
  line L918 (-48.8494, 92.4904) -> (-44.5192, 89.9904)
  line L919 (-44.5192, 89.9904) -> (-40.1891, 92.4904)
  line L920 (-40.1891, 92.4904) -> (-40.1891, 97.4904)
  line L921 (-40.1891, 97.4904) -> (-44.5192, 99.9904)
  line L922 (-34.359, 99.9904) -> (-38.6891, 97.4904)
  line L923 (-38.6891, 97.4904) -> (-38.6891, 92.4904)
  line L924 (-38.6891, 92.4904) -> (-34.359, 89.9904)
  line L925 (-34.359, 89.9904) -> (-30.0289, 92.4904)
  line L926 (-30.0289, 92.4904) -> (-30.0289, 97.4904)
  line L927 (-30.0289, 97.4904) -> (-34.359, 99.9904)
  line L928 (-24.1987, 99.9904) -> (-28.5289, 97.4904)
  line L929 (-28.5289, 97.4904) -> (-28.5289, 92.4904)
  line L930 (-28.5289, 92.4904) -> (-24.1987, 89.9904)
  line L931 (-24.1987, 89.9904) -> (-19.8686, 92.4904)
  line L932 (-19.8686, 92.4904) -> (-19.8686, 97.4904)
  line L933 (-19.8686, 97.4904) -> (-24.1987, 99.9904)
  line L934 (-14.0385, 99.9904) -> (-18.3686, 97.4904)
  line L935 (-18.3686, 97.4904) -> (-18.3686, 92.4904)
  line L936 (-18.3686, 92.4904) -> (-14.0385, 89.9904)
  line L937 (-14.0385, 89.9904) -> (-9.7083, 92.4904)
  line L938 (-9.7083, 92.4904) -> (-9.7083, 97.4904)
  line L939 (-9.7083, 97.4904) -> (-14.0385, 99.9904)
  line L940 (-69.9199, 108.7894) -> (-74.25, 106.2894)
  line L941 (-74.25, 106.2894) -> (-74.25, 101.2894)
  line L942 (-74.25, 101.2894) -> (-69.9199, 98.7894)
  line L943 (-69.9199, 98.7894) -> (-65.5897, 101.2894)
  line L944 (-65.5897, 101.2894) -> (-65.5897, 106.2894)
  line L945 (-65.5897, 106.2894) -> (-69.9199, 108.7894)
  line L946 (-59.7596, 108.7894) -> (-64.0897, 106.2894)
  line L947 (-64.0897, 106.2894) -> (-64.0897, 101.2894)
  line L948 (-64.0897, 101.2894) -> (-59.7596, 98.7894)
  line L949 (-59.7596, 98.7894) -> (-55.4295, 101.2894)
  line L950 (-55.4295, 101.2894) -> (-55.4295, 106.2894)
  line L951 (-55.4295, 106.2894) -> (-59.7596, 108.7894)
  line L952 (-49.5994, 108.7894) -> (-53.9295, 106.2894)
  line L953 (-53.9295, 106.2894) -> (-53.9295, 101.2894)
  line L954 (-53.9295, 101.2894) -> (-49.5994, 98.7894)
  line L955 (-49.5994, 98.7894) -> (-45.2692, 101.2894)
  line L956 (-45.2692, 101.2894) -> (-45.2692, 106.2894)
  line L957 (-45.2692, 106.2894) -> (-49.5994, 108.7894)
  line L958 (-39.4391, 108.7894) -> (-43.7692, 106.2894)
  line L959 (-43.7692, 106.2894) -> (-43.7692, 101.2894)
  line L960 (-43.7692, 101.2894) -> (-39.4391, 98.7894)
  line L961 (-39.4391, 98.7894) -> (-35.109, 101.2894)
  line L962 (-35.109, 101.2894) -> (-35.109, 106.2894)
  line L963 (-35.109, 106.2894) -> (-39.4391, 108.7894)
  line L964 (-29.2789, 108.7894) -> (-33.609, 106.2894)
  line L965 (-33.609, 106.2894) -> (-33.609, 101.2894)
  line L966 (-33.609, 101.2894) -> (-29.2789, 98.7894)
  line L967 (-29.2789, 98.7894) -> (-24.9487, 101.2894)
  line L968 (-24.9487, 101.2894) -> (-24.9487, 106.2894)
  line L969 (-24.9487, 106.2894) -> (-29.2789, 108.7894)
  line L970 (-19.1186, 108.7894) -> (-23.4487, 106.2894)
  line L971 (-23.4487, 106.2894) -> (-23.4487, 101.2894)
  line L972 (-23.4487, 101.2894) -> (-19.1186, 98.7894)
  line L973 (-19.1186, 98.7894) -> (-14.7885, 101.2894)
  line L974 (-14.7885, 101.2894) -> (-14.7885, 106.2894)
  line L975 (-14.7885, 106.2894) -> (-19.1186, 108.7894)
  line L976 (-75, 117.5885) -> (-79.3301, 115.0885)
  line L977 (-79.3301, 115.0885) -> (-79.3301, 110.0885)
  line L978 (-79.3301, 110.0885) -> (-75, 107.5885)
  line L979 (-75, 107.5885) -> (-70.6699, 110.0885)
  line L980 (-70.6699, 110.0885) -> (-70.6699, 115.0885)
  line L981 (-70.6699, 115.0885) -> (-75, 117.5885)
  line L982 (-64.8397, 117.5885) -> (-69.1699, 115.0885)
  line L983 (-69.1699, 115.0885) -> (-69.1699, 110.0885)
  line L984 (-69.1699, 110.0885) -> (-64.8397, 107.5885)
  line L985 (-64.8397, 107.5885) -> (-60.5096, 110.0885)
  line L986 (-60.5096, 110.0885) -> (-60.5096, 115.0885)
  line L987 (-60.5096, 115.0885) -> (-64.8397, 117.5885)
  line L988 (-54.6795, 117.5885) -> (-59.0096, 115.0885)
  line L989 (-59.0096, 115.0885) -> (-59.0096, 110.0885)
  line L990 (-59.0096, 110.0885) -> (-54.6795, 107.5885)
  line L991 (-54.6795, 107.5885) -> (-50.3494, 110.0885)
  line L992 (-50.3494, 110.0885) -> (-50.3494, 115.0885)
  line L993 (-50.3494, 115.0885) -> (-54.6795, 117.5885)
  line L994 (-44.5192, 117.5885) -> (-48.8494, 115.0885)
  line L995 (-48.8494, 115.0885) -> (-48.8494, 110.0885)
  line L996 (-48.8494, 110.0885) -> (-44.5192, 107.5885)
  line L997 (-44.5192, 107.5885) -> (-40.1891, 110.0885)
  line L998 (-40.1891, 110.0885) -> (-40.1891, 115.0885)
  line L999 (-40.1891, 115.0885) -> (-44.5192, 117.5885)
  line L1000 (-34.359, 117.5885) -> (-38.6891, 115.0885)
  line L1001 (-38.6891, 115.0885) -> (-38.6891, 110.0885)
  line L1002 (-38.6891, 110.0885) -> (-34.359, 107.5885)
  line L1003 (-34.359, 107.5885) -> (-30.0289, 110.0885)
  line L1004 (-30.0289, 110.0885) -> (-30.0289, 115.0885)
  line L1005 (-30.0289, 115.0885) -> (-34.359, 117.5885)
  line L1006 (-24.1987, 117.5885) -> (-28.5289, 115.0885)
  line L1007 (-28.5289, 115.0885) -> (-28.5289, 110.0885)
  line L1008 (-28.5289, 110.0885) -> (-24.1987, 107.5885)
  line L1009 (-24.1987, 107.5885) -> (-19.8686, 110.0885)
  line L1010 (-19.8686, 110.0885) -> (-19.8686, 115.0885)
  line L1011 (-19.8686, 115.0885) -> (-24.1987, 117.5885)
  line L1012 (-14.0385, 117.5885) -> (-18.3686, 115.0885)
  line L1013 (-18.3686, 115.0885) -> (-18.3686, 110.0885)
  line L1014 (-18.3686, 110.0885) -> (-14.0385, 107.5885)
  line L1015 (-14.0385, 107.5885) -> (-9.7083, 110.0885)
  line L1016 (-9.7083, 110.0885) -> (-9.7083, 115.0885)
  line L1017 (-9.7083, 115.0885) -> (-14.0385, 117.5885)
  line L1018 (-69.9199, 126.3875) -> (-74.25, 123.8875)
  line L1019 (-74.25, 123.8875) -> (-74.25, 118.8875)
  line L1020 (-74.25, 118.8875) -> (-69.9199, 116.3875)
  line L1021 (-69.9199, 116.3875) -> (-65.5897, 118.8875)
  line L1022 (-65.5897, 118.8875) -> (-65.5897, 123.8875)
  line L1023 (-65.5897, 123.8875) -> (-69.9199, 126.3875)
  line L1024 (-59.7596, 126.3875) -> (-64.0897, 123.8875)
  line L1025 (-64.0897, 123.8875) -> (-64.0897, 118.8875)
  line L1026 (-64.0897, 118.8875) -> (-59.7596, 116.3875)
  line L1027 (-59.7596, 116.3875) -> (-55.4295, 118.8875)
  line L1028 (-55.4295, 118.8875) -> (-55.4295, 123.8875)
  line L1029 (-55.4295, 123.8875) -> (-59.7596, 126.3875)
  line L1030 (-49.5994, 126.3875) -> (-53.9295, 123.8875)
  line L1031 (-53.9295, 123.8875) -> (-53.9295, 118.8875)
  line L1032 (-53.9295, 118.8875) -> (-49.5994, 116.3875)
  line L1033 (-49.5994, 116.3875) -> (-45.2692, 118.8875)
  line L1034 (-45.2692, 118.8875) -> (-45.2692, 123.8875)
  line L1035 (-45.2692, 123.8875) -> (-49.5994, 126.3875)
  line L1036 (-39.4391, 126.3875) -> (-43.7692, 123.8875)
  line L1037 (-43.7692, 123.8875) -> (-43.7692, 118.8875)
  line L1038 (-43.7692, 118.8875) -> (-39.4391, 116.3875)
  line L1039 (-39.4391, 116.3875) -> (-35.109, 118.8875)
  line L1040 (-35.109, 118.8875) -> (-35.109, 123.8875)
  line L1041 (-35.109, 123.8875) -> (-39.4391, 126.3875)
  line L1042 (-29.2789, 126.3875) -> (-33.609, 123.8875)
  line L1043 (-33.609, 123.8875) -> (-33.609, 118.8875)
  line L1044 (-33.609, 118.8875) -> (-29.2789, 116.3875)
  line L1045 (-29.2789, 116.3875) -> (-24.9487, 118.8875)
  line L1046 (-24.9487, 118.8875) -> (-24.9487, 123.8875)
  line L1047 (-24.9487, 123.8875) -> (-29.2789, 126.3875)
  line L1048 (-19.1186, 126.3875) -> (-23.4487, 123.8875)
  line L1049 (-23.4487, 123.8875) -> (-23.4487, 118.8875)
  line L1050 (-23.4487, 118.8875) -> (-19.1186, 116.3875)
  line L1051 (-19.1186, 116.3875) -> (-14.7885, 118.8875)
  line L1052 (-14.7885, 118.8875) -> (-14.7885, 123.8875)
  line L1053 (-14.7885, 123.8875) -> (-19.1186, 126.3875)
  line L1054 (-75, 135.1865) -> (-79.3301, 132.6865)
  line L1055 (-79.3301, 132.6865) -> (-79.3301, 127.6865)
  line L1056 (-79.3301, 127.6865) -> (-75, 125.1865)
  line L1057 (-75, 125.1865) -> (-70.6699, 127.6865)
  line L1058 (-70.6699, 127.6865) -> (-70.6699, 132.6865)
  line L1059 (-70.6699, 132.6865) -> (-75, 135.1865)
  line L1060 (-64.8397, 135.1865) -> (-69.1699, 132.6865)
  line L1061 (-69.1699, 132.6865) -> (-69.1699, 127.6865)
  line L1062 (-69.1699, 127.6865) -> (-64.8397, 125.1865)
  line L1063 (-64.8397, 125.1865) -> (-60.5096, 127.6865)
  line L1064 (-60.5096, 127.6865) -> (-60.5096, 132.6865)
  line L1065 (-60.5096, 132.6865) -> (-64.8397, 135.1865)
  line L1066 (-54.6795, 135.1865) -> (-59.0096, 132.6865)
  line L1067 (-59.0096, 132.6865) -> (-59.0096, 127.6865)
  line L1068 (-59.0096, 127.6865) -> (-54.6795, 125.1865)
  line L1069 (-54.6795, 125.1865) -> (-50.3494, 127.6865)
  line L1070 (-50.3494, 127.6865) -> (-50.3494, 132.6865)
  line L1071 (-50.3494, 132.6865) -> (-54.6795, 135.1865)
  line L1072 (-44.5192, 135.1865) -> (-48.8494, 132.6865)
  line L1073 (-48.8494, 132.6865) -> (-48.8494, 127.6865)
  line L1074 (-48.8494, 127.6865) -> (-44.5192, 125.1865)
  line L1075 (-44.5192, 125.1865) -> (-40.1891, 127.6865)
  line L1076 (-40.1891, 127.6865) -> (-40.1891, 132.6865)
  line L1077 (-40.1891, 132.6865) -> (-44.5192, 135.1865)
  line L1078 (-34.359, 135.1865) -> (-38.6891, 132.6865)
  line L1079 (-38.6891, 132.6865) -> (-38.6891, 127.6865)
  line L1080 (-38.6891, 127.6865) -> (-34.359, 125.1865)
  line L1081 (-34.359, 125.1865) -> (-30.0289, 127.6865)
  line L1082 (-30.0289, 127.6865) -> (-30.0289, 132.6865)
  line L1083 (-30.0289, 132.6865) -> (-34.359, 135.1865)
  line L1084 (-24.1987, 135.1865) -> (-28.5289, 132.6865)
  line L1085 (-28.5289, 132.6865) -> (-28.5289, 127.6865)
  line L1086 (-28.5289, 127.6865) -> (-24.1987, 125.1865)
  line L1087 (-24.1987, 125.1865) -> (-19.8686, 127.6865)
  line L1088 (-19.8686, 127.6865) -> (-19.8686, 132.6865)
  line L1089 (-19.8686, 132.6865) -> (-24.1987, 135.1865)
  line L1090 (-14.0385, 135.1865) -> (-18.3686, 132.6865)
  line L1091 (-18.3686, 132.6865) -> (-18.3686, 127.6865)
  line L1092 (-18.3686, 127.6865) -> (-14.0385, 125.1865)
  line L1093 (-14.0385, 125.1865) -> (-9.7083, 127.6865)
  line L1094 (-9.7083, 127.6865) -> (-9.7083, 132.6865)
  line L1095 (-9.7083, 132.6865) -> (-14.0385, 135.1865)